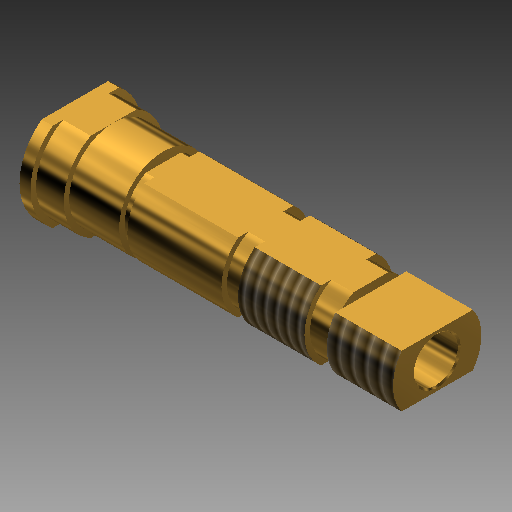
# Autodesk Inventor part: 404-01
Saved by Autodesk Inventor 2019 (Build 230136000, 136)
## iProperties
Company: Autodesk Inc.
Created: 2017-06-27
Part Number: 404-01
Material: Brass, Soft Yellow
Document SubType Name: Modeling
Designer: Autodesk Inc.
Mass: 8.8927 g
Surface Area: 13.6328 cm^2
Volume: 1.04991 cm^3
Density: 8.47 g/cm^3
Appearance: Brass - Satin
Author: Inventor
Autodesk Inventor part; units mm, degrees
ref_plane "YZ Plane" through (0, 0, 0) normal (1, 0, 0) x (0, 1, 0)
ref_plane "XZ Plane" through (0, 0, 0) normal (0, 1, 0) x (-1, 0, 0)
ref_plane "XY Plane" through (0, 0, 0) normal (0, 0, 1) x (1, 0, 0)
sketch "Sketch1" plane through (0, 0, 0) normal (0, 0, 1) x (1, 0, 0)
  line L0 (0, 0) -> (1, 0)
  line L1 (1, 0) -> (1, 5)
  line L2 (1, 5) -> (0, 5)
  line L3 (0, 5) -> (0, 0)
  line L4 (1, 0) -> (3.5, 0)
  line L5 (3.5, 0) -> (3.5, 4.5)
  line L6 (3.5, 4.5) -> (1, 4.5)
  line L7 (1, 4.5) -> (1, 0)
  line L8 (8.75, 0) -> (17.25, 0)
  line L9 (17.25, 0) -> (17.25, 4)
  line L10 (17.25, 4) -> (8.75, 4)
  line L11 (8.75, 4) -> (8.75, 0)
  line L12 (17.25, 0) -> (18.75, 0)
  line L13 (18.75, 0) -> (18.75, 3.5)
  line L14 (18.75, 3.5) -> (17.25, 3.5)
  line L15 (17.25, 3.5) -> (17.25, 0)
  line L16 (18.75, 0) -> (24.75, 0)
  line L17 (24.75, 0) -> (24.75, 4)
  line L18 (24.75, 4) -> (18.75, 4)
  line L19 (18.75, 4) -> (18.75, 0)
  line L20 (24.75, 0) -> (26.75, 0)
  line L21 (26.75, 0) -> (26.75, 3.5)
  line L22 (26.75, 3.5) -> (24.75, 3.5)
  line L23 (24.75, 3.5) -> (24.75, 0)
  line L24 (26.75, 0) -> (32.75, 0)
  line L25 (32.75, 0) -> (32.75, 4)
  line L26 (32.75, 4) -> (26.75, 4)
  line L27 (26.75, 4) -> (26.75, 0)
  line L28 (3.5, 0) -> (8, 0)
  line L29 (8, 0) -> (8, 4)
  line L30 (8, 4) -> (3.5, 4)
  line L31 (3.5, 4) -> (3.5, 0)
  line L32 (8, 0) -> (8.75, 0)
  line L33 (8.75, 0) -> (8.75, 3.5)
  line L34 (8.75, 3.5) -> (8, 3.5)
  line L35 (8, 3.5) -> (8, 0)
  dimension "d0" = 1
  dimension "d1" = 3.5
  dimension "d2" = 32.75
  dimension "d3" = 2
  dimension "d5" = 24.75
  dimension "d6" = 1.5
  dimension "d7" = 17.25
  dimension "d9" = 8
  dimension "d10" = 0.75
  dimension "d11" = 8
  dimension "d12" = 7
  dimension "d13" = 10
  dimension "d14" = 9
  dimension "d15" = 8
  constraints: 72 end point, 18 parallel, 9 horizontal, 9 perpendicular, 4 collinear
  measures "d0" distance of L1.end L2.end
  measures "d1" distance between parallel lines of L5 L3
  measures "d2" distance between parallel lines of L25 L3
  measures "d3" distance of L21.end L22.end
  measures "d5" distance between parallel lines of L17 L3
  measures "d6" distance of L13.end L14.end
  measures "d7" distance between parallel lines of L9 L3
  measures "d9" distance between parallel lines of L29 L3
  measures "d10" distance of L33.end L34.end
  measures "d11" diameter of L26 L24
  measures "d12" diameter of L22 L24
  measures "d13" diameter of L2 L0
  measures "d14" diameter of L6 L4
  measures "d15" diameter of L30 L28
revolve "Revolution1" add sketch "Sketch1" angle 360 about axis through (1, 0, 0) along (1, 0, 0)
thread "Thread1" size "M8x1" class "6g" standard "ANSI Metric M Profile" full length
thread "Thread2" size "M8x1.25" class "6g" standard "ANSI Metric M Profile" full length
sketch "Sketch2" plane through (0, 0, 0) normal (0, 0, 1) x (1, 0, 0)
  line L0 (32.75, 2.375) -> (26.75, 2.375)
  line L1 (26.75, 2.375) -> (26.75, 3.125)
  line L2 (26.75, 3.125) -> (8, 3.125)
  line L3 (8, 3.125) -> (8, 5)
  line L4 (8, 5) -> (32.75, 5)
  line L5 (32.75, 5) -> (32.75, 2.375)
  line L6 (0, 4) -> (4, 4)
  line L7 (4, 4) -> (4, 5)
  line L8 (4, 5) -> (0, 5)
  line L9 (0, 5) -> (0, 4)
  point P0 (0, 0)
  dimension "d21" = 4
  dimension "d22" = 4
  dimension "d23" = 1
  dimension "d24" = 2.375
  dimension "d25" = 32.75
  dimension "d26" = 3.125
  dimension "d27" = 8
  dimension "d28" = 26.75
  constraints: 20 end point, 6 parallel, 2 horizontal, 2 perpendicular, 1 collinear, 1 vertical alignment
  measures "d21" distance from line of L6 point (0, 0)
  measures "d22" distance of L7.end L8.end
  measures "d23" distance of L8.end L6.start
  measures "d24" distance from line of point (0, 0) L0
  measures "d25" distance from line of L5 point (0, 0)
  measures "d26" distance from line of point (0, 0) L2
  measures "d27" distance from line of point (0, 0) L3
  measures "d28" distance from line of point (0, 0) L1
extrude "Extrusion1" cut sketch "Sketch2" along normal mid plane 10
mirror "Mirror1" about plane through (0, 0, 0) normal (0, 1, 0) of "Extrusion1"
hole "Hole1" at (0, 0, 0) direction (1, 0, 0) diameter 4 end through all
chamfer "Chamfer1" distance 0.125 angle 45 1 edges at (32.75, 0, -2)
body "Solid1"
